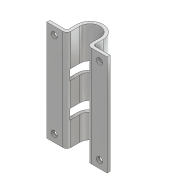
# Autodesk Inventor part: Part1
Saved by Autodesk Inventor 2017 (Build 210142000, 142)
## iProperties
Created: 2023-11-15
Part Number: Part1
Material: Generic
Document SubType Name: Modeling
Designer: Ok
Density: 1 g/cm^3
Appearance: Default
Author: Ok
Autodesk Inventor part; units mm, degrees
ref_plane "YZ Plane" through (0, 0, 0) normal (1, 0, 0) x (0, 1, 0)
ref_plane "XZ Plane" through (0, 0, 0) normal (0, 1, 0) x (-1, 0, 0)
ref_plane "XY Plane" through (0, 0, 0) normal (0, 0, 1) x (1, 0, 0)
sketch "Sketch1" plane through (0, 0, 0) normal (0, 0, 1) x (1, 0, 0)
  arc A0 (5, 0) -> (0, 5) centre (0, 0) ccw
  arc A1 (6.5, 0) -> (0, 6.5) centre (0, 0) ccw
  line L0 (7, -6.5) -> (15, -6.5)
  line L1 (7.5, -5) -> (15, -5)
  line L2 (15, -5) -> (15, -6.5)
  line L3 (6.5, 0) -> (6.5, -4)
  line L4 (0, 10.9318) -> (0, -12.0627) construction
  line L5 (5, 0) -> (5, -4.5)
  arc A2 (5, -4.5) -> (7, -6.5) centre (7, -4.5) ccw
  arc A3 (6.5, -4) -> (7.5, -5) centre (7.5, -4) ccw
  arc A4 (0, 5) -> (-5, 0) centre (0, 0) ccw
  arc A5 (0, 6.5) -> (-6.5, 0) centre (0, 0) ccw
  line L6 (-7, -6.5) -> (-15, -6.5)
  line L7 (-7.5, -5) -> (-15, -5)
  line L8 (-15, -5) -> (-15, -6.5)
  line L9 (-6.5, 0) -> (-6.5, -4)
  line L10 (-5, 0) -> (-5, -4.5)
  arc A6 (-7, -6.5) -> (-5, -4.5) centre (-7, -4.5) ccw
  arc A7 (-7.5, -5) -> (-6.5, -4) centre (-7.5, -4) ccw
  dimension "d0" = 10
  dimension "d1" = 1.5
  dimension "d4" = 2
  dimension "d5" = 1
  constraints: 22 end point, 16 point on circle, 10 symmetric about line, 8 centre point, 4 tangent, 2 coincident, 2 horizontal, 2 perpendicular, 2 vertical, 4 other
  measures "d0" diameter of A0
  measures "d1" radial gap between concentric circles of A0 A1
  measures "d4" radius of A2
  measures "d5" radius of A3
extrude "Extrusion1" add sketch "Sketch1" along normal mid plane 50
sketch "Sketch2" plane through (7.5, -5, 25) normal (0, 1, 0) x (1, 0, 0)
  circle A0 centre (-18.75, 3.75) radius 1.5
  circle A1 centre (3.75, 3.75) radius 1.5
  line L0 (7.5, 50) -> (7.5, 0) projected
  line L1 (-26.7627, 25) -> (16.6618, 25) construction
  circle A2 centre (-18.75, 46.25) radius 1.5
  circle A3 centre (3.75, 46.25) radius 1.5
  point P0 (-7.5, 25)
  constraints: 4 centre point, 2 end point, 2 symmetric about line, 1 horizontal, 2 other
extrude "Extrusion2" cut sketch "Sketch2" against normal up to next
sketch "Sketch3" plane through (0, 0, 0) normal (1, 0, 0) x (0, 1, 0)
  line L0 (-5, 25) -> (-5, -25) construction
  line L1 (-5, -13) -> (11.6912, -13)
  line L2 (11.6912, -13) -> (11.6912, -8)
  line L3 (11.6912, -8) -> (-5, -8)
  line L4 (-5, 4) -> (11.6912, 4)
  line L5 (11.6912, 4) -> (11.6912, 9)
  line L6 (11.6912, 9) -> (-5, 9)
  line L7 (-5, 4) -> (-5, 9)
  line L8 (-5, -13) -> (-5, -8)
  point P0 (0, 0)
  dimension "d16" = 5
  dimension "d17" = 12
  dimension "d18" = 5
  dimension "d19" = 12
  constraints: 16 end point, 4 point on line, 3 vertical, 1 perpendicular
  measures "d16" distance of L1.end L2.end
  measures "d17" distance from line of L0.end L1
  measures "d18" distance of L4.end L5.end
  measures "d19" distance between parallel lines of L3 L4
extrude "Extrusion3" cut sketch "Sketch3" along normal mid plane 50
sketch "Sketch4" plane through (0, 0, 0) normal (0, 1, 0) x (-1, 0, 0)
  line L0 (2.5, 6.6372) -> (-2.5, 6.6372)
  line L1 (-2.5, 6.6372) -> (-2.5, -10.1613)
  line L2 (-2.5, -10.1613) -> (2.5, -10.1613)
  line L3 (2.5, -10.1613) -> (2.5, 6.6372)
  line L4 (2.5, 6.6372) -> (-2.5, -10.1613) construction
  line L5 (-2.5, 6.6372) -> (2.5, -10.1613) construction
  point P0 (0, 0)
  point P1 (0, -1.7621)
  dimension "d22" = 5
  constraints: 12 end point, 2 midpoint, 2 parallel, 1 horizontal, 1 perpendicular
  measures "d22" distance of L2.end L1.end
extrude "Extrusion4" cut sketch "Sketch4" along normal up to next
body "Solid1"
